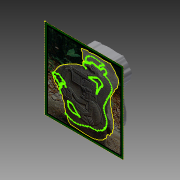
# Autodesk Inventor part: LaVenta
Saved by Autodesk Inventor 2015 (Build 190159000, 159)
## iProperties
Created: 2016-12-02
Part Number: LaVenta
Material: Generic
Document SubType Name: Modeling
Designer: thomas.simms.1
Density: 1 g/cm^3
Appearance: Default
Author: thomas.simms.1
Autodesk Inventor part; units mm, degrees
ref_plane "YZ Plane" through (0, 0, 0) normal (1, 0, 0) x (0, 1, 0)
ref_plane "XZ Plane" through (0, 0, 0) normal (0, 1, 0) x (-1, 0, 0)
ref_plane "XY Plane" through (0, 0, 0) normal (0, 0, 1) x (1, 0, 0)
sketch "Sketch1" plane through (0, 0, 0) normal (0, 0, 1) x (1, 0, 0)
  line L0 (0, 0) -> (150.8125, 0) construction
  line L1 (150.8125, 0) -> (150.8125, -155.575) construction
  line L2 (150.8125, -155.575) -> (0, -155.575) construction
  line L3 (0, -155.575) -> (0, 0) construction
  spline S0 degree 4 poles (118.4391, -131.086) (119.2294, -137.1699) (115.4062, -134.5689) (113.4544, -140.7509) (109.8627, -142.5284) (105.2339, -144.1979) (103.7691, -146.207) (97.2721, -146.6068) (95.376, -148.6526) (88.2903, -148.7496) (83.7659, -148.5562) (75.3991, -149.0693) (69.7531, -147.8341) (65.038, -148.0603) (57.9299, -146.8297) (50.9672, -147.6057) (46.0817, -145.473) (43.2542, -140.5374) (42.3334, -133.3242) (38.8424, -131.2345) (39.4173, -127.4158) (37.0158, -123.2727) (36.5749, -119.9924) (37.3551, -114.7175) (34.6365, -113.6008) (33.6487, -110.934) (33.1173, -108.4248) (33.4381, -104.1531) (29.5601, -102.1885) (28.2456, -100.3973) (24.5599, -99.5465) (24.8226, -96.089) (23.2148, -93.2097) (17.8805, -92.4143) (19.2458, -88.3416) (15.3808, -84.7578) (16.0117, -82.1901) (14.9479, -77.6123) (17.5038, -74.7457) (18.6595, -72.6817) (23.2256, -67.2029) (25.5529, -61.4273) (34.9847, -54.2485) (43.0116, -50.1266) (48.3272, -46.1285) (56.6898, -43.4633) (60.9865, -38.8103) (70.5411, -38.822) (72.35, -37.1464) knots 0 0 0 0 0 0.048471 0.06668 0.084952 0.104017 0.123258 0.143274 0.164958 0.188057 0.21247 0.2364 0.260904 0.284944 0.308524 0.332679 0.356708 0.378711 0.399693 0.419903 0.438728 0.458203 0.477095 0.494602 0.51115 0.527447 0.544724 0.562171 0.579668 0.59639 0.612707 0.630072 0.647841 0.666595 0.685167 0.703761 0.722206 0.73947 0.758265 0.778748 0.803386 0.831787 0.860627 0.888616 0.913927 0.938486 1 1 1 1 1
  spline S1 degree 4 poles (72.35, -37.1464) (72.5908, -35.4167) (72.0973, -33.9104) (71.5944, -29.9173) (76.8228, -28.4875) (73.3743, -27.4896) (71.8728, -26.6292) (72.5171, -23.8671) (72.2026, -22.5864) (72.478, -19.0891) (71.9782, -17.7432) (73.2642, -14.6956) (69.0855, -15.0661) (69.7892, -8.7302) (72.166, -9.3878) (75.2486, -9.0934) (77.6178, -8.2692) (79.3571, -8.6979) (81.3221, -6.7517) (83.5336, -8.7577) (85.7811, -9.417) (87.8256, -7.6072) (90.9213, -8.8834) (92.0848, -6.7711) (95.6219, -7.9819) (98.0079, -6.7819) (103.6061, -7.8747) (105.2812, -7.0016) (109.6539, -8.5331) (112.058, -8.078) (114.6645, -8.2638) (116.8901, -8.1304) (119.7664, -7.1491) (122.4836, -9.8576) (125.5068, -4.4344) (127.1182, -10.0892) (128.3363, -9.8765) knots 0 0 0 0 0 0.069862 0.09665 0.12232 0.146707 0.171141 0.197165 0.223282 0.249044 0.275709 0.303733 0.332126 0.362201 0.392129 0.418692 0.4451 0.470697 0.496102 0.522726 0.550183 0.576629 0.603737 0.631875 0.662782 0.694958 0.728564 0.761399 0.791135 0.820471 0.84837 0.875583 0.903031 0.930285 1 1 1 1 1
  spline S2 degree 4 poles (118.4391, -131.086) (120.0025, -130.6872) (118.1864, -124.851) (127.3756, -131.0184) (124.8362, -121.846) (129.6315, -123.489) (129.2802, -117.2029) (131.0633, -114.2831) (131.4945, -111.1671) (131.2766, -108.6209) (131.5098, -104.8854) (131.0263, -102.2261) (131.1288, -99.1328) (131.2327, -96.6127) (129.645, -93.5253) (129.6146, -92.0068) (128.5056, -86.7691) (126.5924, -85.3911) (128.063, -80.2143) (125.8736, -77.8786) (125.5105, -75.3352) (125.6394, -70.3179) (125.657, -68.985) (125.4968, -64.6729) (125.9818, -62.4778) (128.2975, -58.3338) (130.4088, -56.1791) (130.2595, -52.4965) (134.1055, -50.3305) (133.0421, -47.8687) (135.3014, -45.1653) (136.6986, -44.0979) (139.4498, -40.931) (139.4937, -39.1955) (140.3478, -34.169) (140.757, -32.7045) (142.4319, -28.2033) (140.6463, -26.5463) (140.8836, -23.9282) (138.1532, -22.3472) (136.5955, -21.0934) (136.2386, -19.1559) (134.9666, -17.3971) (134.2987, -14.3306) (130.6054, -13.4893) (130.9797, -12.1679) (128.3363, -9.8765) knots 0 0 0 0 0 0.053098 0.075209 0.099155 0.123475 0.146933 0.170537 0.193245 0.215077 0.237055 0.259047 0.280399 0.300894 0.322683 0.344695 0.367963 0.392022 0.414727 0.43865 0.460626 0.483034 0.505453 0.527865 0.551384 0.574874 0.598838 0.620936 0.642559 0.663209 0.683854 0.704729 0.726889 0.749404 0.772278 0.794913 0.815735 0.836703 0.855947 0.874703 0.893321 0.9112 0.929272 0.947398 1 1 1 1 1
  point P0 (0, 0)
  point P1 (116.9726, -136.0733)
  point P2 (114.6252, -137.8319)
  point P3 (112.278, -140.7645)
  point P4 (109.6369, -142.5236)
  point P5 (105.8211, -144.2835)
  point P6 (103.1798, -145.7495)
  point P7 (98.1893, -146.9236)
  point P8 (94.9605, -148.097)
  point P9 (89.3825, -148.6848)
  point P10 (83.5108, -148.686)
  point P11 (75.411, -148.6877)
  point P12 (69.712, -148.1022)
  point P13 (65.0145, -147.8099)
  point P14 (57.9684, -147.2245)
  point P15 (50.9222, -146.9325)
  point P16 (46.5182, -144.8792)
  point P17 (43.5818, -139.8905)
  point P18 (41.3569, -133.4703)
  point P19 (39.5498, -130.6784)
  point P20 (38.8838, -127.5639)
  point P21 (37.4159, -123.4543)
  point P22 (36.8289, -119.3444)
  point P23 (36.4288, -114.9917)
  point P24 (34.8685, -113.1845)
  point P25 (33.801, -111.1366)
  point P26 (33.3071, -108.4808)
  point P27 (32.5696, -104.6001)
  point P28 (29.7852, -102.0205)
  point P29 (27.7308, -100.5518)
  point P30 (25.3828, -99.0828)
  point P31 (24.5024, -96.44)
  point P32 (22.7415, -93.797)
  point P33 (19.2195, -91.7404)
  point P34 (18.2403, -88.5375)
  point P35 (16.1874, -84.7586)
  point P36 (15.6973, -81.8837)
  point P37 (15.6973, -77.7704)
  point P38 (17.1647, -75.0067)
  point P39 (18.632, -72.9528)
  point P40 (21.8608, -68.5502)
  point P41 (25.9703, -62.3862)
  point P42 (35.1856, -54.5711)
  point P43 (43.5836, -49.4702)
  point P44 (49.0427, -46.2512)
  point P45 (54.1507, -43.895)
  point P46 (59.1405, -41.2545)
  point P47 (66.7728, -38.9067)
  point P48 (72.3436, -34.7284)
  point P49 (72.3375, -32.1633)
  point P50 (73.9534, -29.5987)
  point P51 (75.382, -28.4382)
  point P52 (73.7149, -27.4984)
  point P53 (72.327, -26.3266)
  point P54 (72.3235, -24.2247)
  point P55 (72.3208, -22.3557)
  point P56 (72.3196, -19.3116)
  point P57 (72.3188, -17.4384)
  point P58 (72.3189, -15.5634)
  point P59 (70.3281, -14.0983)
  point P60 (70.3288, -9.8825)
  point P61 (72.3296, -9.214)
  point P62 (75.3831, -8.9306)
  point P63 (77.7102, -8.4918)
  point P64 (79.3542, -8.2497)
  point P65 (81.2329, -7.5381)
  point P66 (83.5064, -8.466)
  point P67 (85.6937, -8.9261)
  point P68 (88.0409, -8.215)
  point P69 (90.6221, -8.2075)
  point P70 (92.2647, -7.4999)
  point P71 (94.9717, -7.4947)
  point P72 (98.2028, -7.2565)
  point P73 (103.195, -7.4873)
  point P74 (105.8371, -7.4875)
  point P75 (109.6535, -8.1904)
  point P76 (112.2939, -8.1939)
  point P77 (114.6401, -8.199)
  point P78 (116.9851, -7.9723)
  point P79 (119.6759, -7.7467)
  point P80 (121.7825, -8.2204)
  point P81 (124.1192, -7.2973)
  point P82 (126.2262, -8.0045)
  point P83 (119.6632, -128.923)
  point P84 (121.7697, -127.5773)
  point P85 (125.2738, -127.0904)
  point P86 (126.2173, -123.4789)
  point P87 (128.3242, -122.1504)
  point P88 (129.7281, -117.7036)
  point P89 (130.9107, -113.8876)
  point P90 (131.365, -111.1686)
  point P91 (131.3639, -108.5295)
  point P92 (131.3634, -105.0083)
  point P93 (131.1389, -102.0483)
  point P94 (131.1289, -99.1377)
  point P95 (130.8951, -96.4947)
  point P96 (129.9588, -93.8503)
  point P97 (129.4911, -91.7932)
  point P98 (128.3216, -87.4788)
  point P99 (127.2884, -84.7818)
  point P100 (127.2898, -80.494)
  point P101 (126.2196, -77.8029)
  point P102 (125.6231, -75.0191)
  point P103 (125.6245, -70.6777)
  point P104 (125.6254, -68.555)
  point P105 (125.6265, -65.1781)
  point P106 (126.2328, -62.3836)
  point P107 (128.3448, -58.6007)
  point P108 (129.9874, -55.783)
  point P109 (131.1538, -52.6505)
  point P110 (133.2724, -50.0069)
  point P111 (133.6981, -47.8182)
  point P112 (135.1408, -45.4863)
  point P113 (136.7894, -43.8599)
  point P114 (138.8987, -41.2169)
  point P115 (139.6013, -38.8691)
  point P116 (140.3037, -34.6779)
  point P117 (141.0054, -32.1031)
  point P118 (141.7069, -28.3576)
  point P119 (141.0024, -26.252)
  point P120 (140.2976, -24.1471)
  point P121 (138.188, -22.2742)
  point P122 (136.7874, -20.8694)
  point P123 (136.0775, -19.2314)
  point P124 (135.138, -17.3617)
  point P125 (134.1984, -15.4923)
  point P126 (132.557, -14.0888)
  point P127 (131.1499, -12.919)
  point P128 (0, 0)
  constraints: 1 coincident, 136 other
extrude "Extrusion1" add sketch "Sketch1" along normal mid plane 25.4
sketch "Sketch2" plane through (0, 0, 12.7) normal (0, 0, 1) x (1, 0, 0)
  point P0 (0, 0)
sketch "Sketch3" plane through (0, 0, 12.7) normal (0, 0, 1) x (1, 0, 0)
  line L0 (0, 0) -> (150.8125, 0) construction
  line L1 (150.8125, 0) -> (150.8125, -155.575) construction
  line L2 (150.8125, -155.575) -> (0, -155.575) construction
  line L3 (0, -155.575) -> (0, 0) construction
  spline S0 degree 4 poles (78.7767, -26.7441) (78.7679, -23.6404) (79.3504, -23.1194) (79.8294, -18.0894) (83.8562, -16.5981) (85.5709, -14.8201) (89.5043, -13.554) (93.3789, -13.2748) (94.5075, -12.7337) (104.7717, -14.5606) (105.446, -14.0761) (113.2341, -15.5061) (114.131, -15.8271) knots 0 0 0 0 0 0.193487 0.266944 0.34549 0.424519 0.500523 0.586181 0.672442 0.764154 1 1 1 1 1
  spline S1 degree 4 poles (114.131, -15.8271) (113.1236, -17.0174) (112.4309, -17.3501) (109.9706, -18.949) (108.2962, -19.2029) (106.5674, -21.0073) (105.1546, -20.6438) (104.7586, -23.6769) (105.2294, -24.8127) knots 0 0 0 0 0 0.324635 0.446172 0.561686 0.673185 1 1 1 1 1
  spline S2 degree 3 poles (105.2294, -24.8127) (105.0472, -24.3731) (103.525, -25.0373) (101.9256, -24.852) (99.9557, -24.2212) (97.8664, -24.1737) (96.0077, -22.8013) (93.847, -23.6658) (92.0989, -22.244) (90.4373, -23.3028) (88.966, -23.8165) (87.5345, -24.9125) (87.2591, -26.0483) (87.0904, -26.7441) knots 0 0 0 0 0.142761 0.319112 0.54319 0.739236 0.938847 1.18238 1.344566 1.522509 1.699061 1.830237 2.037644 2.037644 2.037644 2.037644
  spline S3 degree 4 poles (78.7767, -26.7441) (79.8322, -26.312) (82.0455, -26.5743) (84.3428, -26.1344) (86.2651, -26.1448) (87.0904, -26.7441) knots 0 0 0 0 0 0.514865 1 1 1 1 1
  spline S4 degree 4 poles (79.7844, -37.7635) (79.6014, -37.1891) (75.8742, -38.6662) (76.0293, -36.3871) (74.494, -35.4065) (74.5848, -33.646) (74.7684, -31.6339) (75.5389, -30.1814) (77.3814, -30.0153) (79.0847, -29.4608) (80.4279, -28.9198) (81.8818, -28.4839) (83.0062, -27.9908) (85.0897, -27.7583) (87.1697, -26.9662) (88.0011, -27.6158) (87.8462, -25.8972) knots 0 0 0 0 0 0.162136 0.222411 0.283695 0.346366 0.412236 0.479473 0.543728 0.607525 0.66887 0.728954 0.790948 0.851345 1 1 1 1 1
  spline S5 degree 4 poles (87.8462, -25.8972) (88.4512, -26.0008) (88.2097, -23.7734) (90.4371, -24.6611) (90.9739, -23.1935) (92.1724, -23.5876) (93.3635, -23.5198) (94.1301, -24.0497) (95.289, -24.2222) (96.0514, -24.9522) (97.5384, -25.2773) (98.8282, -25.1877) (100.4942, -25.6179) (101.7076, -25.8857) (103.3045, -26.2326) (104.7046, -26.6267) (106.1164, -26.0201) (107.428, -27.1828) (109.0105, -26.1996) (109.0902, -23.925) (110.6952, -24.3796) (111.5838, -22.2978) (112.4844, -22.7059) (113.1822, -22.1254) knots 0 0 0 0 0 0.100105 0.140722 0.181016 0.219911 0.259874 0.299989 0.340922 0.384156 0.429908 0.477091 0.525031 0.573003 0.619843 0.666947 0.71389 0.761966 0.807766 0.852751 0.895817 1 1 1 1 1
  spline S6 degree 4 poles (113.1822, -22.1254) (113.9529, -21.4375) (114.4161, -22.3925) (116.9634, -21.7326) (117.5976, -23.7616) (118.5747, -24.1131) (118.6495, -25.355) (118.7914, -26.1959) (118.5652, -27.5191) (118.0919, -27.5892) (117.5422, -28.6455) (116.9812, -28.7264) (116.9199, -30.5975) (115.7411, -30.3027) (115.2534, -31.1679) (115.1278, -31.2253) knots 0 0 0 0 0 0.191307 0.269042 0.344217 0.415424 0.484479 0.549666 0.613906 0.673655 0.733823 0.797288 0.860584 1 1 1 1 1
  spline S7 degree 4 poles (115.3838, -120.4749) (116.0263, -119.327) (118.3883, -117.4384) (118.1828, -113.4168) (119.4791, -109.8009) (119.4211, -106.9991) (118.6491, -103.9566) (118.2044, -101.2749) (117.1495, -99.0365) (115.5393, -96.2666) (114.6082, -93.5803) (114.1642, -91.212) (113.4894, -88.2797) (113.6694, -86.4329) (113.8404, -82.8632) (115.5259, -80.8456) (116.7823, -77.5333) (118.1049, -75.1959) (119.8728, -71.3501) (120.3011, -68.4222) (123.2493, -65.386) (123.7513, -62.233) (125.9237, -59.2013) (126.7073, -55.7712) (128.6075, -53.156) (129.4041, -48.9625) (128.9318, -46.4338) (127.7067, -41.1406) (125.3302, -40.0048) (122.989, -36.1476) (118.381, -33.1367) (116.3526, -33.4102) (115.4629, -31.6214) (115.1278, -31.2253) knots 0 0 0 0 0 0.073384 0.103743 0.134054 0.163518 0.192558 0.222125 0.251408 0.280543 0.309868 0.337768 0.365961 0.394543 0.423884 0.454474 0.485995 0.518037 0.550689 0.583648 0.616205 0.648957 0.681222 0.714017 0.746374 0.779931 0.812985 0.846932 0.882335 0.914796 0.945087 1 1 1 1 1
  spline S8 degree 4 poles (67.6075, -124.6107) (66.1918, -124.5903) (64.8922, -124.8337) (63.6307, -124.5371) (61.0498, -124.6331) (59.4571, -124.589) (57.605, -124.6564) (56.2704, -124.4833) (53.6022, -125.0413) (52.3847, -123.4352) (50.0725, -122.7897) (48.5365, -122.1161) (47.3101, -120.4492) (46.0209, -119.7625) (45.8889, -118.5859) (45.5146, -116.7631) (44.9455, -115.4113) (44.7671, -112.6211) (44.8647, -111.2941) (45.1016, -110.7234) knots 0 0 0 0 0 0.130407 0.180688 0.232734 0.285662 0.340326 0.395939 0.453753 0.512777 0.570576 0.625388 0.675484 0.724833 0.771561 0.821449 0.875157 1 1 1 1 1
  spline S9 degree 4 poles (67.6075, -124.6107) (65.881, -124.0041) (65.9616, -122.8525) (62.6041, -122.8895) (62.7622, -120.5238) (60.8786, -120.5063) (60.7342, -119.486) (59.6139, -118.6138) (59.6483, -117.6973) (58.1703, -116.9961) (57.8633, -116.0217) (56.4636, -115.1091) (55.8234, -113.6893) (54.6419, -112.2747) (53.2604, -111.9424) (52.3746, -110.3329) (50.4825, -110.6434) (49.1678, -110.5704) (47.4864, -110.5273) (46.0635, -110.057) (45.1766, -110.476) (45.1016, -110.7234) knots 0 0 0 0 0 0.138782 0.188254 0.234642 0.279213 0.32209 0.364907 0.408397 0.45318 0.501753 0.552203 0.604135 0.656304 0.708363 0.759164 0.809753 0.859862 0.906852 1 1 1 1 1
  spline S10 degree 4 poles (85.7468, -50.6857) (86.8177, -50.35) (86.4634, -50.3673) (87.7733, -49.1826) (88.9074, -49.22) (89.4685, -48.3695) (90.7371, -48.2576) (91.2545, -47.7414) (92.217, -47.3972) (92.7463, -46.9397) (94.4403, -47.1073) (94.5113, -45.9386) (95.9647, -45.9838) (96.262, -45.1934) (97.5601, -45.1314) (98.4274, -44.3916) (99.5184, -44.0457) (100.7043, -43.9042) (101.8542, -43.6892) (103.0683, -44.1491) (104.7404, -44.4511) (105.951, -45.2617) (107.0393, -45.3423) (107.9433, -46.1548) (108.6804, -46.6919) (109.3499, -47.1845) (110.0547, -47.8115) (110.1874, -48.3625) (110.4078, -49.257) (112.0069, -49.2531) (110.6861, -50.1514) (111.1918, -50.457) knots 0 0 0 0 0 0.076632 0.106954 0.140025 0.171655 0.20331 0.234523 0.266465 0.29893 0.332233 0.365209 0.397206 0.43036 0.463878 0.49916 0.534531 0.570319 0.608288 0.647307 0.686189 0.724355 0.759484 0.792417 0.824409 0.853926 0.881948 0.909522 0.935106 1 1 1 1 1
  spline S11 degree 4 poles (100.4334, -69.9806) (100.7438, -68.9487) (100.7286, -67.9236) (101.3975, -66.7406) (102.6021, -65.0909) (103.0762, -64.0511) (103.2624, -63.0089) (103.673, -61.9028) (104.8446, -61.1038) (105.2579, -60.1138) (105.5076, -59.0807) (106.1034, -58.0484) (106.6167, -56.9843) (107.5026, -56.0077) (107.9219, -55.0256) (108.6527, -54.3644) (110.0333, -53.8085) (111.0393, -52.8075) (109.7389, -51.2958) (112.1758, -51.3016) (111.1918, -50.457) knots 0 0 0 0 0 0.136358 0.188713 0.240458 0.291401 0.341728 0.391623 0.441567 0.49158 0.54107 0.59185 0.642577 0.692403 0.743327 0.792169 0.840572 0.888899 1 1 1 1 1
  spline S12 degree 4 poles (100.4334, -69.9806) (100.4443, -69.1272) (100.4025, -67.7552) (100.4844, -66.8266) (100.3385, -64.7683) (100.8162, -63.6833) (100.8053, -60.5982) (100.647, -59.6013) (101.148, -55.9217) (100.6285, -55.6635) (101.7786, -52.0447) (98.936, -53.0777) (97.434, -52.2528) (96.6458, -52.6454) (94.6728, -51.7852) (94.2989, -52.1196) (92.8662, -51.7853) (91.1524, -52.5244) (91.0009, -50.8749) (89.5701, -51.3851) (88.609, -51.179) (87.3994, -51.3251) (86.5759, -51.3658) (85.7468, -50.6857) knots 0 0 0 0 0 0.104676 0.145195 0.190838 0.239977 0.294256 0.347979 0.400202 0.452742 0.501304 0.548942 0.594817 0.634905 0.674026 0.715221 0.75379 0.794617 0.832923 0.868107 0.903157 1 1 1 1 1
  spline S13 degree 4 poles (40.8341, -132.6848) (41.6284, -133.3095) (43.1804, -133.7671) (44.8861, -135.805) (47.8163, -136.8671) (50.651, -137.9041) (53.2861, -138.4038) (56.7451, -139.5914) (59.3846, -139.0574) (62.4227, -139.5593) (65.8259, -138.4811) (69.0364, -138.4797) (72.3249, -135.7566) (75.309, -136.7061) (79.1002, -134.5412) (81.8568, -134.1093) (84.3371, -132.5366) (88.1108, -131.9407) (90.7433, -132.3314) (93.4236, -132.6102) (97.5303, -130.999) (101.3257, -132.5831) (103.4352, -129.4439) (109.8434, -126.7478) (111.4371, -126.2502) (114.3383, -122.1774) (115.3838, -120.4749) knots 0.019 0.019 0.019 0.019 0.019 0.081259 0.11584 0.151731 0.189055 0.226525 0.26398 0.302192 0.340339 0.379935 0.419812 0.460387 0.500217 0.538935 0.578369 0.615855 0.652927 0.691791 0.730594 0.770603 0.813622 0.854735 0.89563 1 1 1 1 1
  spline S14 degree 4 poles (15.5777, -78.4716) (16.438, -78.5406) (17.1652, -76.6035) (18.2723, -74.988) (20.6421, -74.7006) (21.7698, -76.3837) (23.7367, -75.8033) (25.084, -75.187) (26.4229, -73.6703) (29.072, -75.0559) (30.2182, -75.837) (30.7549, -77.3368) (33.6843, -77.7174) (33.7459, -79.0407) (35.9774, -79.4926) (34.9511, -80.7107) knots 0 0 0 0 0 0.164713 0.232949 0.299285 0.365473 0.433355 0.505387 0.576621 0.646625 0.716989 0.780992 0.844682 1 1 1 1 1
  line L4 (34.6964, -127.8581) -> (46.9718, -137.5116) construction
  arc A0 (39.5262, -129.3746) -> (44.3593, -133.1754) centre (43.0172, -129.9088) ccw construction
  spline S15 degree 4 poles (34.9511, -80.7107) (35.3648, -80.2552) (35.5605, -80.3337) (36.1459, -80.0962) (36.9331, -80.5189) (37.2868, -80.818) (37.6454, -81.1827) (38.0912, -81.2967) (38.3994, -81.5973) (38.8975, -81.6583) (38.8882, -82.0105) (38.975, -82.6384) (38.8837, -82.9569) (38.8538, -83.5902) (38.8541, -83.9872) (38.8874, -84.7247) (38.4992, -84.6785) (37.8945, -84.8717) (37.6378, -84.6993) (36.9488, -84.5826) (36.9474, -85.4477) (35.8767, -85) (35.4352, -85.7968) (34.7068, -85.6083) (33.9789, -85.8364) (33.7582, -86.467) (32.6867, -86.5794) (32.2177, -87.0051) (31.5064, -86.9184) (31.7603, -88.4619) (31.5883, -89.2123) (31.57, -90.1642) (31.7743, -91.9396) (30.7247, -90.7586) (29.5093, -92.3154) (28.9626, -91.0694) (28.1513, -91.7769) knots 0 0 0 0 0 0.064408 0.089274 0.115102 0.140588 0.16488 0.188265 0.210309 0.233177 0.255923 0.279874 0.305513 0.330833 0.355443 0.379967 0.403363 0.426346 0.450638 0.476271 0.504292 0.533554 0.563576 0.592738 0.622818 0.652663 0.681287 0.712137 0.743326 0.777531 0.814668 0.848649 0.882126 0.913848 1 1 1 1 1
  spline S16 degree 4 poles (28.1513, -91.7769) (28.4873, -91.7179) (27.466, -90.5735) (28.202, -90.2818) (28.3264, -89.0752) (27.4894, -88.7798) (26.6738, -88.6676) (26.0581, -88.4168) (24.9583, -88.3053) (24.5192, -87.8277) (24.7218, -87.1217) (24.5919, -86.1297) (24.7905, -85.4403) (23.6643, -85.9093) (22.9947, -85.2633) (22.2783, -85.5931) (21.6498, -85.2078) (21.2296, -85.0441) (20.9533, -83.9697) (20.2709, -83.5753) (20.6337, -82.9381) (20.2981, -81.6284) (20.9062, -80.3184) (19.2905, -81.5532) (18.6594, -81.8238) (17.987, -83.0398) (15.3371, -81.4974) (17.9341, -81.1799) (15.0236, -78.3004) (15.5777, -78.4716) knots 0 0 0 0 0 0.074374 0.107138 0.139453 0.1725 0.207269 0.240796 0.273522 0.307538 0.337981 0.369795 0.402793 0.434011 0.466612 0.497554 0.528803 0.559849 0.59065 0.626239 0.660482 0.696956 0.736223 0.773881 0.81435 0.852585 0.894547 1 1 1 1 1
  spline S17 degree 4 poles (31.0631, -102.9828) (31.2548, -101.9361) (30.276, -100.7858) (30.0199, -100.0922) (29.2476, -98.4817) (28.8818, -97.4855) (29.0701, -96.3739) (28.8526, -95.2213) (30.4674, -95.3712) (30.1128, -94.6663) (29.8922, -93.9407) (31.2039, -93.1628) (31.4464, -94.1367) (32.5239, -93.5042) (31.8839, -92.7525) (32.6989, -91.7289) (32.2774, -91.0264) (32.3976, -90.1576) (32.6995, -88.8709) (32.1477, -88.0866) (33.4361, -87.7908) (33.9708, -87.4844) (34.6297, -86.5422) (35.7522, -86.1019) (36.2505, -85.5818) (37.6363, -85.4125) (39.3525, -85.3619) (39.48, -87.6529) (40.6708, -86.7903) (40.8341, -87.7961) knots 0 0 0 0 0 0.10044 0.137166 0.174326 0.21134 0.247201 0.279505 0.309545 0.340403 0.36983 0.40039 0.431038 0.461816 0.493168 0.526021 0.561424 0.59482 0.628773 0.662032 0.694324 0.72893 0.763177 0.799705 0.836851 0.874404 0.912147 1 1 1 1 1
  point P0 (79.1126, -23.2171)
  point P1 (79.7844, -20.8658)
  point P2 (81.296, -18.0945)
  point P3 (83.5634, -16.499)
  point P4 (85.7468, -15.0714)
  point P5 (89.6097, -13.7277)
  point P6 (92.8848, -13.2239)
  point P7 (94.8163, -13.0559)
  point P8 (100.9466, -13.8117)
  point P9 (105.2294, -14.3156)
  point P10 (110.52, -15.0714)
  point P11 (112.7034, -17.1708)
  point P12 (111.1918, -18.0945)
  point P13 (109.4283, -18.9343)
  point P14 (108.2526, -19.4382)
  point P15 (107.0769, -20.278)
  point P16 (106.0692, -20.8658)
  point P17 (105.2295, -22.1255)
  point P18 (103.8018, -24.8127)
  point P19 (102.0383, -24.8127)
  point P20 (99.8549, -24.3088)
  point P21 (97.9234, -23.9729)
  point P22 (96.0759, -23.2171)
  point P23 (93.6406, -23.2171)
  point P24 (92.129, -22.6293)
  point P25 (90.4495, -23.2171)
  point P26 (88.8539, -23.9729)
  point P27 (87.8462, -24.8127)
  point P28 (80.5275, -26.4278)
  point P29 (82.3841, -26.3679)
  point P30 (84.1808, -26.2482)
  point P31 (85.7468, -26.2482)
  point P32 (76.0705, -37.2512)
  point P33 (75.4071, -36.2255)
  point P34 (74.7884, -35.3281)
  point P35 (74.5961, -33.789)
  point P36 (74.9168, -31.6723)
  point P37 (75.7505, -30.4534)
  point P38 (77.3539, -29.9399)
  point P39 (79.1135, -29.4265)
  point P40 (80.5283, -28.9131)
  point P41 (81.8434, -28.4639)
  point P42 (82.9978, -28.0788)
  point P43 (84.5371, -27.7578)
  point P44 (86.3971, -27.3727)
  point P45 (87.4873, -27.1801)
  point P46 (88.4014, -25.2349)
  point P47 (89.2718, -24.3088)
  point P48 (90.4495, -23.9729)
  point P49 (91.115, -23.4941)
  point P50 (92.1291, -23.4941)
  point P51 (93.3166, -23.6477)
  point P52 (94.187, -23.9729)
  point P53 (95.1598, -24.3088)
  point P54 (96.0759, -24.8126)
  point P55 (97.4126, -25.1837)
  point P56 (98.8462, -25.2861)
  point P57 (100.4334, -25.5932)
  point P58 (101.7646, -25.8972)
  point P59 (103.3006, -26.2481)
  point P60 (104.7342, -26.4277)
  point P61 (106.0692, -26.3679)
  point P62 (107.4478, -26.7441)
  point P63 (108.7278, -25.8972)
  point P64 (109.4282, -24.3088)
  point P65 (110.2126, -23.9729)
  point P66 (111.1918, -23.2171)
  point P67 (112.107, -22.6293)
  point P68 (114.1309, -21.8556)
  point P69 (115.4349, -22.1253)
  point P70 (116.9709, -22.6291)
  point P71 (117.7901, -23.6476)
  point P72 (118.4046, -24.3087)
  point P73 (118.6606, -25.286)
  point P74 (118.7118, -26.3679)
  point P75 (118.4559, -27.3726)
  point P76 (118.0974, -27.7574)
  point P77 (117.5342, -28.463)
  point P78 (117.1246, -28.9119)
  point P79 (116.7663, -29.9383)
  point P80 (116.1006, -30.4514)
  point P81 (115.3838, -30.9693)
  point P82 (116.76, -118.5849)
  point P83 (118.089, -115.7429)
  point P84 (118.6998, -112.4755)
  point P85 (119.2803, -109.724)
  point P86 (119.2773, -106.9705)
  point P87 (118.6902, -103.928)
  point P88 (118.0733, -101.3442)
  point P89 (117.0968, -99.046)
  point P90 (115.6524, -96.2281)
  point P91 (114.6758, -93.5239)
  point P92 (114.108, -91.0405)
  point P93 (113.6559, -88.4435)
  point P94 (113.6577, -86.3296)
  point P95 (114.118, -83.2561)
  point P96 (115.3753, -80.7119)
  point P97 (116.7628, -77.7966)
  point P98 (118.0989, -75.0827)
  point P99 (119.6221, -71.4904)
  point P100 (120.7782, -68.4503)
  point P101 (122.8003, -65.2932)
  point P102 (124.071, -62.2766)
  point P103 (125.6577, -59.1032)
  point P104 (126.926, -55.9323)
  point P105 (128.3516, -52.9223)
  point P106 (129.1419, -49.2806)
  point P107 (128.8221, -46.1157)
  point P108 (127.394, -41.8456)
  point P109 (125.4885, -39.627)
  point P110 (122.4746, -36.2121)
  point P111 (118.7172, -33.7768)
  point P112 (116.7718, -32.9768)
  point P113 (115.6796, -31.9847)
  point P114 (65.5161, -124.6802)
  point P115 (64.2663, -124.6802)
  point P116 (62.947, -124.6108)
  point P117 (61.1416, -124.6108)
  point P118 (59.4057, -124.6107)
  point P119 (57.7392, -124.6107)
  point P120 (56.2116, -124.6107)
  point P121 (53.9201, -124.6107)
  point P122 (52.1842, -123.6386)
  point P123 (50.1011, -122.7359)
  point P124 (48.504, -121.8332)
  point P125 (47.1153, -120.4748)
  point P126 (46.2126, -119.6112)
  point P127 (45.8654, -118.5769)
  point P128 (45.5182, -116.9726)
  point P129 (45.1711, -115.7275)
  point P130 (44.8933, -113.7091)
  point P131 (44.8933, -111.6955)
  point P132 (65.7073, -123.4837)
  point P133 (64.2663, -122.736)
  point P134 (62.947, -121.8333)
  point P135 (62.3167, -120.8011)
  point P136 (61.1416, -120.2608)
  point P137 (60.5469, -119.5156)
  point P138 (59.8223, -118.577)
  point P139 (59.4057, -117.8059)
  point P140 (58.4336, -116.9727)
  point P141 (57.7392, -116.1395)
  point P142 (56.6976, -115.0979)
  point P143 (55.7255, -113.7092)
  point P144 (54.5451, -112.4536)
  point P145 (53.3647, -111.6955)
  point P146 (52.1842, -110.7234)
  point P147 (50.5234, -110.574)
  point P148 (49.1041, -110.574)
  point P149 (47.7537, -110.4637)
  point P150 (46.3481, -110.287)
  point P151 (45.3835, -110.4637)
  point P152 (86.6781, -50.2772)
  point P153 (87.0776, -49.9144)
  point P154 (88.0372, -49.3353)
  point P155 (88.8332, -49.0557)
  point P156 (89.5851, -48.5311)
  point P157 (90.6593, -48.1513)
  point P158 (91.3439, -47.7735)
  point P159 (92.1025, -47.3923)
  point P160 (92.8597, -47.0844)
  point P161 (94.1662, -46.808)
  point P162 (94.7981, -46.1701)
  point P163 (95.7774, -45.8019)
  point P164 (96.3907, -45.3748)
  point P165 (97.4067, -45.0216)
  point P166 (98.4574, -44.4786)
  point P167 (99.5277, -44.0903)
  point P168 (100.673, -43.8952)
  point P169 (101.7684, -43.8179)
  point P170 (103.0353, -44.0865)
  point P171 (104.7343, -44.5878)
  point P172 (106.0656, -45.1674)
  point P173 (107.0687, -45.5205)
  point P174 (107.9749, -46.1539)
  point P175 (108.7128, -46.7168)
  point P176 (109.4102, -47.2569)
  point P177 (109.9875, -47.8692)
  point P178 (110.1971, -48.3946)
  point P179 (110.5072, -48.9223)
  point P180 (111.1756, -49.3307)
  point P181 (111.1839, -49.7883)
  point P182 (100.776, -68.465)
  point P183 (101.1174, -67.3953)
  point P184 (101.7646, -66.2709)
  point P185 (102.5728, -65.0344)
  point P186 (103.0324, -64.0039)
  point P187 (103.3006, -63.025)
  point P188 (103.8018, -61.9945)
  point P189 (104.7342, -61.0156)
  point P190 (105.2294, -60.0881)
  point P191 (105.5611, -59.1199)
  point P192 (106.0691, -58.0787)
  point P193 (106.6946, -56.9967)
  point P194 (107.4478, -55.9496)
  point P195 (107.9866, -55.0904)
  point P196 (108.7275, -54.4206)
  point P197 (110.0063, -53.6992)
  point P198 (110.5197, -52.9389)
  point P199 (110.5197, -51.999)
  constraints: 2 end point, 2 midpoint, 1 centre point, 1 point on circle, 400 other
body "Solid1"
